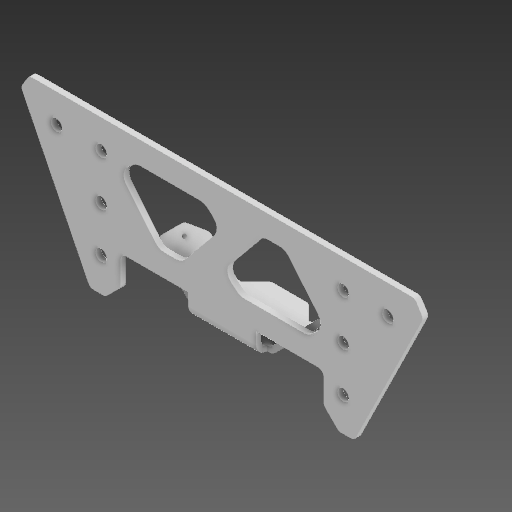
# Autodesk Inventor part: SpineChestConnector
Saved by Autodesk Inventor 2020 (Build 240168000, 168)
## iProperties
Created: 2020-05-06
Part Number: SpineChestConnector
Material: Generic
Document SubType Name: Sheet Metal
Designer: valer
Density: 1 g/cm^3
Sheet Metal Rule: Default
Appearance: Default
Flat Pattern Width: 10.621 cm
Flat Pattern Length: 22.5304 cm
Flat Pattern Area: 239.296 cm^2
Sheet Metal Width: 4.182 in
Sheet Metal Length: 8.870 in
Sheet Metal Area: 37.091 in^2
Author: valer
Autodesk Inventor part; units mm, degrees
ref_plane "YZ Plane" through (0, 0, 0) normal (1, 0, 0) x (0, 1, 0)
ref_plane "XZ Plane" through (0, 0, 0) normal (0, 1, 0) x (-1, 0, 0)
ref_plane "XY Plane" through (0, 0, 0) normal (0, 0, 1) x (1, 0, 0)
sketch "Base" plane through (0, 0, 0) normal (0, 0, 1) x (1, 0, 0)
  circle A0 centre (-93.1394, 0) radius 3.175
  circle A1 centre (-68.0201, 0) radius 3.175
  circle A2 centre (-68.0201, -25.4) radius 3.175
  circle A3 centre (-68.0201, -50.8) radius 3.175
  circle A4 centre (68.0201, -25.4) radius 3.175
  circle A5 centre (68.0201, 0) radius 3.175
  circle A6 centre (68.0201, -50.8) radius 3.175
  circle A7 centre (93.1394, 0) radius 3.175
  line L0 (116.8584, 16.3476) -> (74.2804, -69.7602)
  line L1 (-116.8584, 16.3476) -> (-74.2804, -69.7602)
  line L2 (-116.8584, 16.3476) -> (116.8584, 16.3476)
  line L3 (-74.2804, -69.7602) -> (74.2804, -69.7602)
  line L4 (-93.1394, 0) -> (-68.0201, 0) construction
  line L5 (68.0201, 0) -> (93.1394, 0) construction
  line L6 (68.0201, 0) -> (68.0201, -50.8) construction
  line L7 (-68.0201, 0) -> (-68.0201, -50.8) construction
  line L8 (-68.0201, 0) -> (68.0201, 0) construction
  line L9 (0, 16.3476) -> (0, -69.7602) construction
  line L10 (-57.15, -69.7602) -> (-57.15, -44.3602)
  line L11 (-57.15, -44.3602) -> (57.15, -44.3602)
  line L12 (57.15, -44.3602) -> (57.15, -69.7602)
  line L13 (0, -44.3602) -> (0, -69.7602) construction
  line L14 (-19.05, -44.3602) -> (19.05, -44.3602)
  line L15 (19.05, -44.3602) -> (19.05, -57.0602)
  line L16 (19.05, -57.0602) -> (-19.05, -57.0602)
  line L17 (-19.05, -57.0602) -> (-19.05, -44.3602)
  point P0 (0, 0)
  point P1 (136.6687, 223.6471)
  point P2 (0, 0)
  point P3 (0, -57.0602)
  dimension "d0" = 233.7169
  dimension "d1" = 86.1079
  dimension "d2" = 63.689
  dimension "d3" = 63.689
  dimension "d4" = 6.35
  dimension "d5" = 16.3476
  dimension "d6" = 14.0157
  dimension "d7" = 14.0157
  dimension "d8" = 50.8
  dimension "d9" = 25.1193
  dimension "d10" = 114.3
  dimension "d11" = 25.4
  dimension "d55" = 38.1
  dimension "d56" = 12.7
  measures "d0" distance of L1.start L0.start
  measures "d1" vertical distance of L1.start L1.end
  measures "d2" angle of L2 L1
  measures "d3" angle of L2 L0
  measures "d4" diameter of A0
  measures "d5" distance between parallel lines of L2 L8
  measures "d6" distance from line of L1 L4.start
  measures "d7" distance from line of L0 L5.end
  measures "d8" distance of L5.start L6.end
  measures "d9" distance of L5.start L5.end
  measures "d10" distance of L10.end L11.end
  measures "d11" distance of L10.start L10.end
  measures "d55" distance of L15.end L16.end
  measures "d56" distance of L16.end L14.start
extrude "Plate1" add sketch "Base" along normal blind 3.048 contours L0 L3 L12 L11 L10 L1 L2 | L15 L16 L17 L11
sketch "Sketch2" plane through (-19.05, -54.0122, 3.048) normal (0, -1, 0) x (1, 0, 0)
  line L0 (38.1, 0) -> (0, 0)
  line L1 (0, 0) -> (0, -38.1)
  line L2 (0, -38.1) -> (38.1, -38.1)
  line L3 (38.1, -38.1) -> (38.1, 0)
  constraints: 6 end point, 1 horizontal, 1 perpendicular, 1 vertical
edge flange "SpineMountFlangeFeature" height 38.1 angle 90 thickness 3.048 bend radius 3.048 thickness toward (0, -1, 0) relief straight relief width 3.048 relief depth 1.524 edges at (0, -57.0602, 0) wall of the first edge with corners at (19.05, -54.0122, 3.048) (-19.05, -54.0122, 3.048) (-19.05, -54.0122, -35.052) (19.05, -54.0122, -35.052)
bend "Bend1"
corner "Corner1"
chamfer "FlangeChamferFeature" distance 8.4667 angle 45 6 edges at (-57.15, -69.7602, 1.524) (57.15, -69.7602, 1.524) (116.8584, 16.3476, 1.524) (-116.8584, 16.3476, 1.524) (-19.05, -55.5362, -35.052) (19.05, -55.5362, -35.052)
sketch "GenerativeCut" plane through (0, 0, 3.048) normal (0, 0, 1) x (1, 0, 0)
  line L0 (-57.953, -4.5158) -> (-35.5242, -31.6602)
  line L1 (-35.5242, -31.6602) -> (-22.8242, -31.6602)
  line L2 (-22.8242, -31.6602) -> (-0.3954, -4.5158)
  line L3 (-0.3954, -4.5158) -> (-10.1242, 3.6476)
  line L4 (-10.1242, 3.6476) -> (-48.2242, 3.6476)
  line L5 (-48.2242, 3.6476) -> (-57.953, -4.5158)
  line L6 (0.3954, -23.4968) -> (22.8242, 3.6476)
  line L7 (0.3954, -23.4968) -> (10.1242, -31.6602)
  line L8 (10.1242, -31.6602) -> (48.2242, -31.6602)
  line L9 (48.2242, -31.6602) -> (57.953, -23.4968)
  line L10 (57.953, -23.4968) -> (35.5242, 3.6476)
  line L11 (35.5242, 3.6476) -> (22.8242, 3.6476)
  line L12 (-108.3918, 16.3476) -> (108.3918, 16.3476) projected
  circle A0 centre (-68.0201, 0) radius 3.175 projected
  circle A1 centre (68.0201, -25.4) radius 3.175 projected
  line L13 (57.15, -44.3602) -> (19.05, -44.3602) projected
  point P0 (0, 0)
  dimension "d26" = 12.7
  dimension "d27" = 140
  dimension "d28" = 12.7
  dimension "d30" = 12.7
  dimension "d32" = 140
  dimension "d33" = 140
  dimension "d34" = 140
  dimension "d35" = 38.1
  dimension "d36" = 10.0671
  dimension "d37" = 10.0671
  dimension "d57" = 12.7
  constraints: 24 end point, 7 equal length, 3 parallel, 2 collinear, 1 horizontal
  measures "d26" distance between parallel lines of L6 L2
  measures "d27" angle of L9 L8
  measures "d28" distance between parallel lines of L12 L4
  measures "d30" distance of L10.end L6.end
  measures "d32" angle of L7 L8
  measures "d33" angle of L3 L4
  measures "d34" angle of L4 L5
  measures "d35" distance of L7.end L8.end
  measures "d36" horizontal distance of L0.start A0.centre
  measures "d37" horizontal distance of A1.centre L9.end
  measures "d57" distance between parallel lines of L13 L8
extrude "GenerativeCutFeature" cut sketch "GenerativeCut" against normal blind 25.4 contours L5 L4 L3 L2 L1 L0 | L6 L11 L10 L9 L8 L7
fillet "GenerativeFilletsFeature" radius 6.35 12 edges at (-57.953, -4.5158, 1.524) (-48.2242, 3.6476, 1.524) (-10.1242, 3.6476, 1.524) (-0.3954, -4.5158, 1.524) (-35.5242, -31.6602, 1.524) (-22.8242, -31.6602, 1.524) (0.3954, -23.4968, 1.524) (10.1242, -31.6602, 1.524) (22.8242, 3.6476, 1.524) (35.5242, 3.6476, 1.524) (57.953, -23.4968, 1.524) (48.2242, -31.6602, 1.524)
sketch "Sketch6" plane through (-19.05, -57.0602, -3.048) normal (0, -1, 0) x (1, 0, 0)
  line L0 (0, -23.5373) -> (0, 0)
  line L1 (0, -23.5373) -> (-3.175, -23.5373)
  line L2 (-3.175, -23.5373) -> (-3.175, 0)
  line L3 (-3.175, 0) -> (0, 0)
  line L4 (0, 0) -> (0, -23.5373)
  line L5 (38.1, 0) -> (0, 0) construction
  line L6 (19.05, 0) -> (19.05, -32.004) construction
  line L7 (29.6333, -32.004) -> (8.4667, -32.004) construction
  line L8 (38.1, -23.5373) -> (38.1, 0)
  line L9 (38.1, -23.5373) -> (41.275, -23.5373)
  line L10 (41.275, -23.5373) -> (41.275, 0)
  line L11 (41.275, 0) -> (38.1, 0)
  point P0 (19.05, 3.048)
  dimension "d58" = 3.175
  measures "d58" distance of L0.start L1.end
sheet face with bend "MountExtendFeature" sketch "Sketch6" thickness 3.048 toward (0, 1, 0) bend radius 3.048 relief straight relief width 3.048 relief depth 1.524 contours L1 L2 L3 L0
bend "Bend3"
mirror "MirrorFeature" about plane through (0, 0, 0) normal (1, 0, 0) of "MountExtendFeature"
sketch "Sketch7" plane through (-20.0697, -54.905, -3.048) normal (-0.7071068, -0.7071068, 0) x (0.7071068, -0.7071068, 0)
  line L0 (0, -23.5373) -> (0, 0)
  line L1 (0, 0) -> (-31.75, 0)
  line L2 (-31.75, 0) -> (-31.75, -23.5373)
  line L3 (-31.75, -23.5373) -> (0, -23.5373)
  constraints: 6 end point, 1 horizontal, 1 perpendicular, 1 vertical
edge flange "SideFlangsFeature" height 31.75 angle 45 thickness 3.048 bend radius 3.048 thickness toward (-0.7071068, -0.7071068, 0) relief straight relief width 3.048 relief depth 1.524 corner gap 3.048 corner form 0 edges at (-22.225, -54.0122, -14.8167) (22.225, -54.0122, -14.8167) wall of the first edge with corners at (-20.0697, -54.905, -26.5853) (-20.0697, -54.905, -3.048) (-42.5204, -32.4543, -3.048) (-42.5204, -32.4543, -26.5853)
bend "Bend4"
corner "Corner3"
sketch "FrontHoles" plane through (-10.5833, -57.0602, -35.052) normal (0, -1, 0) x (1, 0, 0)
  circle A0 centre (16.9333, 20.2353) radius 1.27
  circle A1 centre (4.2333, 20.2353) radius 1.27
  point P0 (10.5833, 35.052)
  constraints: 2 centre point
sketch "RightHoles" plane through (44.6756, -34.6096, -3.048) normal (0.7071068, -0.7071068, 0) x (-0.7071068, -0.7071068, 0)
  ellipse E0 centre (13.4934, 11.7687) end of major axis (13.4934, 13.0387) minor radius 1.2652
  ellipse E1 centre (5.059, 11.7687) end of major axis (5.059, 13.0387) minor radius 1.2652
  point P0 (7.1178, -3.048)
  constraints: 4 other
sketch "LeftHoles" plane through (-44.6756, -34.6096, -3.048) normal (-0.7071068, -0.7071068, 0) x (-0.7071068, 0.7071068, 0)
  ellipse E0 centre (-13.4934, 11.7687) end of major axis (-13.4934, 13.0387) minor radius 1.2652
  ellipse E1 centre (-5.059, 11.7687) end of major axis (-5.059, 13.0387) minor radius 1.2652
  point P0 (-7.1178, -3.048)
  constraints: 2 centre point
hole "FrontHolesFeature" at (-6.35, -57.0602, -14.8167) at (6.35, -57.0602, -14.8167) direction (0, 1, 0) diameter 2.54 end through all
hole "LeftHolesFeature" at (-41.0984, -38.1868, -14.8167) at (-35.1343, -44.1509, -14.8167) direction (0.7071068, 0.7071068, 0) diameter 2.54 end through all
hole "RightHolesFeature" at (35.1343, -44.1509, -14.8167) at (41.0984, -38.1868, -14.8167) direction (-0.7071068, 0.7071068, 0) diameter 2.54 end through all
chamfer "MountChamferFeature" distance 8.4667 angle 45 2 edges at (-43.598, -33.532, -26.5853) (43.598, -33.532, -26.5853)
fillet "OutsideFilletsFeature" radius 3.175 12 edges at (-108.3918, 16.3476, 1.524) (-113.1056, 8.7581, 1.524) (108.3918, 16.3476, 1.524) (113.1056, 8.7581, 1.524) (-57.15, -44.3602, 1.524) (-57.15, -61.2936, 1.524) (-65.6167, -69.7602, 1.524) (-74.2804, -69.7602, 1.524) (57.15, -44.3602, 1.524) (65.6167, -69.7602, 1.524) (74.2804, -69.7602, 1.524) (57.15, -61.2936, 1.524)
fillet "OutsideMountFilletsFeature" radius 3.175 8 edges at (-43.598, -33.532, -18.1187) (-37.6112, -39.5188, -26.5853) (-43.598, -33.532, -3.048) (-10.5833, -55.5362, -35.052) (10.5833, -55.5362, -35.052) (37.6112, -39.5188, -26.5853) (43.598, -33.532, -18.1187) (43.598, -33.532, -3.048)
equation "\"d3\" = d2"
equation "\"d32\" = d27"
equation "\"d33\" = d27"
equation "\"d34\" = d27"
equation "\"d37\" = d36"
equation "\"d79\" = Thickness"
equation "\"d86\" = Thickness"
equation "\"d93\" = Thickness"
equation "\"d12\" = Thickness"
equation "\"d13\" = BendReliefWidth"
equation "\"d14\" = BendReliefDepth"
equation "\"d15\" = MinimumRemnant"
equation "\"d16\" = TransitionRadius"
equation "\"d19\" = BendRadius"
equation "\"d20\" = CornerReliefSize"
equation "\"d21\" = GapSize"
equation "\"d22\" = JacobiRadiusSize"
equation "\"d59\" = BendRadius"
equation "\"d60\" = BendReliefWidth"
equation "\"d62\" = MinimumRemnant"
equation "\"d61\" = BendReliefDepth"
equation "\"d63\" = TransitionRadius"
equation "\"d64\" = BendReliefWidth"
equation "\"d65\" = BendReliefDepth"
equation "\"d66\" = MinimumRemnant"
equation "\"d67\" = TransitionRadius"
equation "\"d70\" = BendRadius"
equation "\"d71\" = CornerReliefSize"
equation "\"d72\" = GapSize"
equation "\"d73\" = JacobiRadiusSize"
equation "\"BendRadius\" = Thickness"
equation "\"BendReliefWidth\" = Thickness"
equation "\"BendReliefDepth\" = 0.5 * Thickness"
equation "\"CornerReliefSize\" = 4 * Thickness"
equation "\"MinimumRemnant\" = 2 * Thickness"
equation "\"TransitionRadius\" = BendRadius"
equation "\"JacobiRadiusSize\" = BendRadius"
equation "\"GapSize\" = Thickness"
equation "\"Thickness\" = 3.048"
body "Solid1"
